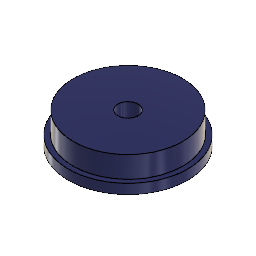
4-Roller_End_Cap v2 v3 (Autodesk Fusion 360 design; units mm, degrees)
Autodesk Fusion 360 part; units mm, degrees
sketch "Roller_End_Cap_Outter" plane through (0, 0, 0) normal (0, 0, 1) x (1, 0, 0)
  circle A0 centre (0, 0) radius 38.1
  dimension "d2" = 76.2
  constraint coincident A0.centre origin
  measures "d2" diameter of A0
extrude "Extrude1" add sketch "Roller_End_Cap_Outter" along normal blind 6.35
sketch "Roller_End_Cap_Inner" plane through (0, 0, 6.35) normal (0, 0, 1) x (-1, 0, 0)
  circle A0 centre (0, 0) radius 38.1
  circle A1 centre (0, 0) radius 34.925
  dimension "d7" = 69.85
  constraint coincident A0.centre A1.centre
  measures "d7" diameter of A1
extrude "Extrude3" add sketch "Roller_End_Cap_Inner" along normal blind 10 contours A1
sketch "Shaft Hole" plane through (0, 0, 16.35) normal (0, 0, 1) x (-1, 0, 0)
  circle A0 centre (0, 0) radius 34.925
  circle A1 centre (0, 0) radius 6.45
  dimension "d10" = 12.9
  constraint concentric A0 A1
  measures "d10" diameter of A1
extrude "Extrude4" cut sketch "Shaft Hole" against normal through all contours A1
extrude "Extrude5" add 1 faces at (-25.3033, 1.7351, 16.35) along direction (0, 0, 1) blind 3.65
named bodies: "Roller_End_Cap"
